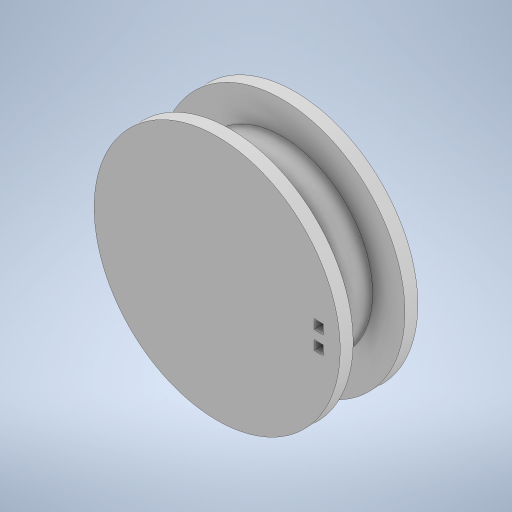
# Autodesk Inventor part: spool
Saved by Autodesk Inventor 2023 (Build 270158000, 158)
## iProperties
Created: 2022-10-02
Part Number: spool
Material: Generic
Document SubType Name: Modeling
Designer: carso
Density: 1 g/cm^3
Appearance: Default
Author: carso
Autodesk Inventor part; units mm, degrees
ref_plane "YZ Plane" through (0, 0, 0) normal (1, 0, 0) x (0, 1, 0)
ref_plane "XZ Plane" through (0, 0, 0) normal (0, 1, 0) x (-1, 0, 0)
ref_plane "XY Plane" through (0, 0, 0) normal (0, 0, 1) x (1, 0, 0)
sketch "Sketch1" plane through (0, 0, 0) normal (0, 0, 1) x (1, 0, 0)
  circle A0 centre (0, 0) radius 35
  dimension "d0" = 70
  constraints: 1 centre point, 1 coincident
  measures "d0" diameter of A0
extrude "Extrusion1" add sketch "Sketch1" along normal blind 20
sketch "Sketch2" plane through (0, 0, 20) normal (0, 0, 1) x (1, 0, 0)
  circle A0 centre (0, 0) radius 47.5
  dimension "d3" = 95
  constraints: 1 centre point, 1 coincident
  measures "d3" diameter of A0
extrude "Extrusion2" add sketch "Sketch2" along normal blind 5
sketch "Sketch3" plane through (0, 0, 0) normal (0, 0, -1) x (-1, 0, 0)
  circle A0 centre (0, 0) radius 47.5
  dimension "d6" = 95
  constraints: 1 centre point, 1 coincident
  measures "d6" diameter of A0
extrude "Extrusion3" add sketch "Sketch3" along normal blind 5
sketch "Sketch4" plane through (0, 0, -5) normal (0, 0, -1) x (-1, 0, 0)
  circle A0 centre (0, 0) radius 2.65
  line L0 (-2.65, 0) -> (2.03, 0)
  line L1 (2.03, 0) -> (2.03, -1.7034)
  line L2 (2.03, 0) -> (2.03, 1.7034)
  dimension "d9" = 5.3
  dimension "d10" = 4.68
  constraints: 6 end point, 3 point on circle, 1 centre point, 1 coincident, 1 horizontal, 1 perpendicular, 1 point on line
  measures "d9" diameter of A0
  measures "d10" distance of L0.start L0.end
extrude "Extrusion4" cut sketch "Sketch4" against normal blind 21 contours L2 L0 A0 | A0 L0 L1
extrude "Extrusion5" cut sketch "Sketch4" against normal blind 4 contours A0 L1 L2
sketch "Sketch5" plane through (0, 0, 25) normal (0, 0, 1) x (1, 0, 0)
  line L0 (57.5, 1.75) -> (37.5, 1.75)
  line L1 (37.5, 1.75) -> (37.5, -1.75)
  line L2 (37.5, -1.75) -> (57.5, -1.75)
  line L3 (57.5, -1.75) -> (57.5, 1.75)
  circle A0 centre (0, 0) radius 47.5 projected
  line L4 (57.5, 1.75) -> (37.5, -1.75) construction
  line L5 (37.5, 1.75) -> (57.5, -1.75) construction
  line L6 (41, 5.25) -> (37.5, 5.25)
  line L7 (37.5, 5.25) -> (37.5, -5.25)
  line L8 (37.5, -5.25) -> (41, -5.25)
  line L9 (41, -5.25) -> (41, 5.25)
  point P0 (47.5, 0)
  point P1 (37.5, 0)
  point P2 (41, -1.75)
  point P3 (41, 1.75)
  point P4 (47.4678, 1.75)
  point P5 (47.4678, -1.75)
  dimension "d15" = 20
  dimension "d16" = 3.5
  dimension "d21" = 3.5
  dimension "d22" = 3.5
  dimension "d23" = 3.5
  dimension "d24" = 0
  constraints: 20 end point, 4 parallel, 3 midpoint, 2 horizontal, 2 perpendicular, 2 other
  measures "d15" distance of L0.start L0.end
  measures "d16" distance of L1.end L0.end
  measures "d21" distance between parallel lines of L6 L0
  measures "d22" distance between parallel lines of L8 L2
  measures "d23" distance between parallel lines of L9 L1
  measures "d24" distance between parallel lines of L7 L1
extrude "Extrusion6" cut sketch "Sketch5" against normal blind 10 contours L3 L2 A0 L0 | L0 L7 L6 L9 | L9 L8 L7 L2
equation "\"d6\" = d3"
body "Solid1"
